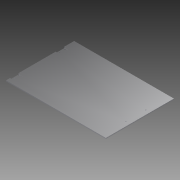
# Autodesk Inventor part: EnclosureDoorFront
Saved by Autodesk Inventor 2015 SP1 (Build 190203100, 203)
## iProperties
Category: Panel
Created: 2015-01-21
Part Number: EnclosureDoorFront
Material: Polycarbonate, Clear
Document SubType Name: Modeling
Designer: Jack
Density: 1.2 g/cm^3
Appearance: Polycarbonate - Clear
Mass: 824.904 g
Surface Area: 3504.94 cm^2
Volume: 687.42 cm^3
Vendor: Tap Plastics
Catalog Web Link: N/A
Author: Jack
Title: Enclosure Door Panel
Autodesk Inventor part; units mm, degrees
ref_plane "YZ Plane" through (0, 0, 0) normal (1, 0, 0) x (0, 1, 0)
ref_plane "XZ Plane" through (0, 0, 0) normal (0, 1, 0) x (-1, 0, 0)
ref_plane "XY Plane" through (0, 0, 0) normal (0, 0, 1) x (1, 0, 0)
sketch "Sketch1" plane through (0, 0, 0) normal (0, 0, 1) x (1, 0, 0)
  line L0 (0, 0) -> (490.75, 0)
  line L1 (490.75, 0) -> (490.75, 335)
  line L2 (490.75, 335) -> (0, 335)
  line L3 (0, 335) -> (0, 0)
  dimension "d0" = 490.75
  dimension "d1" = 335
  constraints: 8 end point, 2 parallel, 1 horizontal, 1 perpendicular
  measures "d0" distance of L2.end L1.end
  measures "d1" distance of L1.end L0.end
extrude "Extrusion1" add sketch "Sketch1" along normal blind 4.7625
sketch "Sketch3" plane through (0, 0, 4.7625) normal (0, 0, 1) x (1, 0, 0)
  line L0 (0, 0) -> (490.75, 0) projected
  line L1 (0, 335) -> (0, 0) projected
  line L2 (0, 61) -> (6, 61)
  line L3 (6, 61) -> (6, 20)
  line L4 (490.75, 335) -> (0, 335) projected
  line L5 (0, 244) -> (6, 244)
  line L6 (6, 244) -> (6, 285)
  line L7 (6, 285) -> (0, 285)
  line L8 (6, 20) -> (0, 20)
  dimension "d11" = 41
  dimension "d12" = 6
  dimension "d15" = 41
  dimension "d16" = 6
  dimension "d27" = 50
  dimension "d28" = 20
  constraints: 12 end point, 4 point on line, 3 horizontal, 3 perpendicular
  measures "d11" distance of L2.end L3.end
  measures "d12" distance of L2.start L2.end
  measures "d15" distance of L5.end L6.end
  measures "d16" distance of L5.start L5.end
  measures "d27" distance between parallel lines of L4 L7
  measures "d28" distance between parallel lines of L0 L8
extrude "Extrusion3" cut sketch "Sketch3" against normal up to next
sketch "Sketch4" plane through (0, 0, 0) normal (0, 0, -1) x (-1, 0, 0)
  line L0 (-6, 244) -> (-6, 285) projected
  line L1 (-490.75, 335) -> (0, 335) projected
  line L2 (0, 0) -> (-490.75, 0) projected
  line L3 (-6, 20) -> (-6, 61) projected
  line L4 (-6, 244) -> (-20.5, 244)
  line L5 (-20.5, 244) -> (-20.5, 285)
  line L6 (-6, 61) -> (-20.5, 61)
  line L7 (-20.5, 61) -> (-20.5, 20)
  line L8 (-6, 285) -> (-20.5, 285)
  line L9 (-20.5, 20) -> (-6, 20)
  point P0 (-6, 335)
  point P1 (-6, 0)
  dimension "d17" = 14.5
  dimension "d18" = 14.5
  constraints: 12 end point, 4 perpendicular, 2 horizontal
  measures "d17" distance of L0.start L4.end
  measures "d18" distance of L3.end L6.end
extrude "Extrusion4" cut sketch "Sketch4" against normal blind 2
sketch "Sketch5" plane through (0, 0, 4.7625) normal (0, 0, 1) x (1, 0, 0)
  line L0 (490.75, 0) -> (490.75, 335) projected
  line L1 (490.75, 335) -> (0, 335) projected
  circle A0 centre (446.75, 217.5) radius 2.5
  circle A1 centre (446.75, 117.5) radius 2.5
  point P0 (6, 335)
  dimension "d21" = 5
  dimension "d22" = 100
  dimension "d23" = 117.5
  dimension "d24" = 44
  constraints: 2 centre point, 1 equal radius, 1 vertical alignment
  measures "d21" diameter of A1
  measures "d22" distance of A0.centre A1.centre
  measures "d23" distance from line of L1 A0.centre
  measures "d24" distance from line of L0 A1.centre
extrude "Extrusion5" cut sketch "Sketch5" against normal up to next
sketch "Sketch6" plane through (0, 0, 2) normal (0, 0, -1) x (-1, 0, 0)
  line L0 (-20.5, 285) -> (-6, 285) projected
  line L1 (-6, 244) -> (-20.5, 244) projected
  line L2 (-6, 61) -> (-6, 20) projected
  line L3 (-20.5, 61) -> (-6, 61) projected
  line L4 (-20.5, 20) -> (-20.5, 61) projected
  line L5 (-6, 20) -> (-20.5, 20) projected
  circle A0 centre (-12, 277) radius 2.75
  circle A1 centre (-12, 252) radius 2.75
  circle A2 centre (-12, 53) radius 2.75
  circle A3 centre (-12, 28) radius 2.75
  point P0 (0, 0)
  dimension "d29" = 5.5
  dimension "d30" = 5.5
  dimension "d31" = 5.5
  dimension "d32" = 5.5
  dimension "d34" = 8
  dimension "d35" = 8
  dimension "d36" = 8.5
  dimension "d37" = 8
  dimension "d38" = 8
  constraints: 4 centre point, 3 vertical alignment
  measures "d29" diameter of A0
  measures "d30" diameter of A1
  measures "d31" diameter of A2
  measures "d32" diameter of A3
  measures "d34" distance from line of L5 A3.centre
  measures "d35" distance from line of L3 A2.centre
  measures "d36" distance from line of L4 A2.centre
  measures "d37" distance from line of L1 A1.centre
  measures "d38" distance from line of L0 A0.centre
extrude "Extrusion6" cut sketch "Sketch6" against normal up to next contours A0 | A1 | A2 | A3
body "Solid1"
